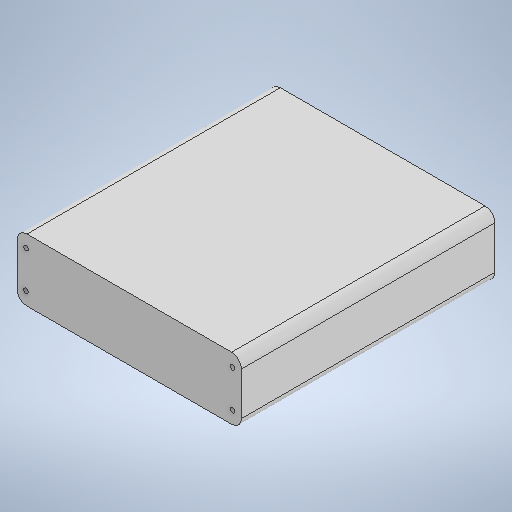
# Autodesk Inventor part: Lardis_grob
Saved by Autodesk Inventor 2025.1 (Build 291241000, 241)
## iProperties
Created: 2024-04-17
Part Number: Lardis_grob
Material: Generisch
Document SubType Name: Modeling
Designer: Holger
Density: 1 g/cm^3
Appearance: Vorgabe
Author: Holger
Autodesk Inventor part; units mm, degrees
ref_plane "YZ Plane" through (0, 0, 0) normal (1, 0, 0) x (0, 1, 0)
ref_plane "XZ Plane" through (0, 0, 0) normal (0, 1, 0) x (-1, 0, 0)
ref_plane "XY Plane" through (0, 0, 0) normal (0, 0, 1) x (1, 0, 0)
sketch "Skizze1" plane through (0, 0, 0) normal (0, 1, 0) x (-1, 0, 0)
  line L0 (52.5, 16) -> (-52.5, 16)
  line L1 (-57.5, 11) -> (-57.5, -11)
  line L2 (-52.5, -16) -> (52.5, -16)
  line L3 (57.5, -11) -> (57.5, 11)
  line L4 (81.9497, 0) -> (-81.9497, 0) projected
  line L5 (0, -23.8497) -> (0, 23.8497) projected
  arc A0 (57.5, 11) -> (52.5, 16) centre (52.5, 11) ccw
  arc A1 (52.5, -16) -> (57.5, -11) centre (52.5, -11) ccw
  arc A2 (-52.5, 16) -> (-57.5, 11) centre (-52.5, 11) ccw
  arc A3 (-57.5, -11) -> (-52.5, -16) centre (-52.5, -11) ccw
  circle A4 centre (53, 9.5) radius 1.5
  circle A5 centre (53, -9.5) radius 1.5
  circle A6 centre (-53, 9.5) radius 1.5
  circle A7 centre (-53, -9.5) radius 1.5
  point P0 (0, 0)
  point P1 (57.5, 16)
  point P2 (-57.5, 16)
  point P3 (57.5, -16)
  dimension "d0" = 115
  dimension "d1" = 32
  dimension "d2" = 5
  dimension "d3" = 3
  dimension "d4" = 9.5
  dimension "d5" = 53
  constraints: 8 centre point, 8 end point, 8 point on circle, 8 tangent, 6 point on line, 3 equal radius, 3 symmetric about line, 2 parallel, 1 horizontal, 1 perpendicular, 5 other
  measures "d0" distance of point (57.5, 16) point (-57.5, 16)
  measures "d1" distance of point (57.5, -16) point (57.5, 16)
  measures "d2" radius of A0
  measures "d3" diameter of A4
  measures "d4" distance from line of A4.centre L4
  measures "d5" distance from line of A4.centre L5
extrude "Extrusion1" add sketch "Skizze1" along normal blind 130 contours A0 L3 L4 L5 L0 | L5 L4 L1 A2 L0 | L5 L2 A3 L1 L4 | L4 L3 A1 L2 L5 | A4 | A5 | A6 | A7
hole "Bohrung1" at (53, 0, 9.5) at (53, 0, -9.5) at (-53, 0, 9.5) at (-53, 0, -9.5) direction (0, 1, 0) diameter 2.459 depth 12 tip angle 118 thread size "M3x0.5" class "6H" standard "ISO Metric profile"
